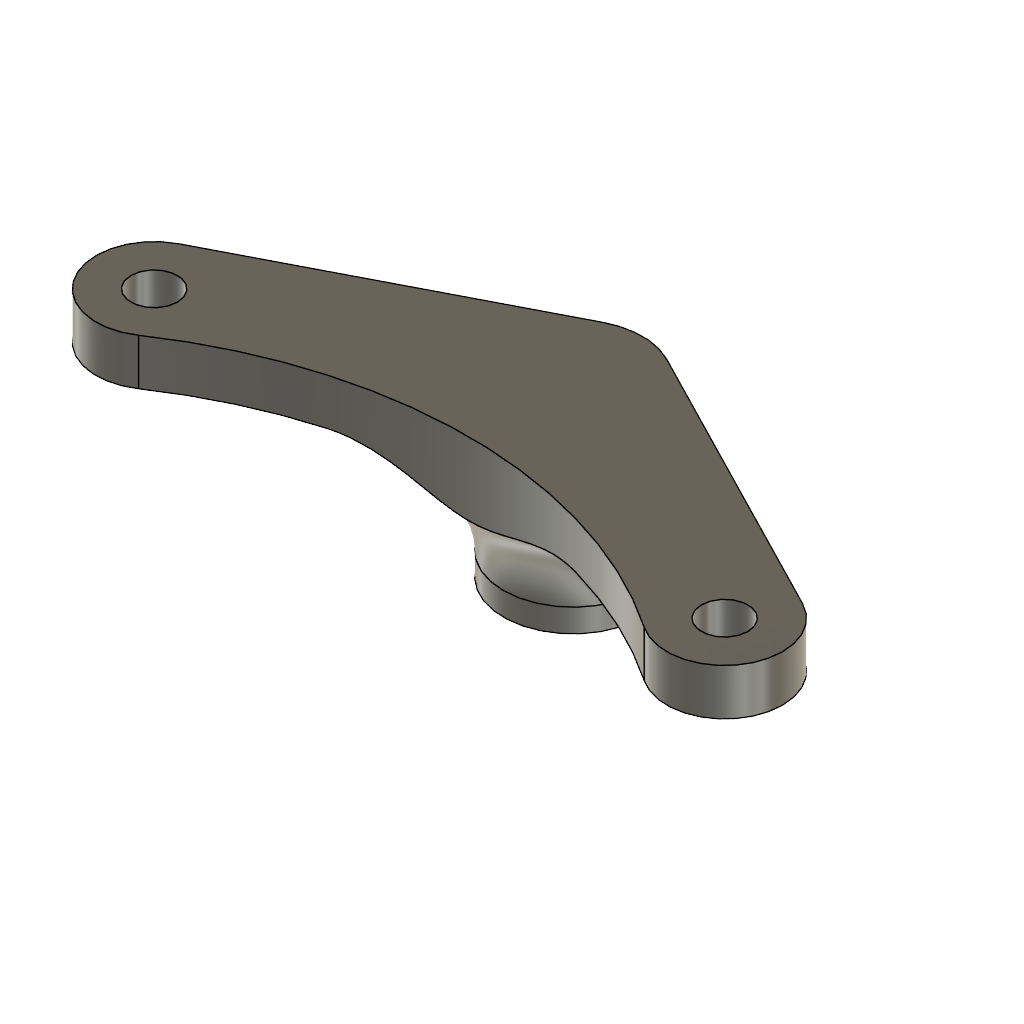
Haltebrücke (Autodesk Fusion 360 design; units mm, degrees)
Autodesk Fusion 360 part; units mm, degrees
sketch "Skizze1" plane through (0, 0, 0) normal (0, 0, 1) x (1, 0, 0)
  circle A0 centre (0, 0) radius 22 construction
  circle A1 centre (-12.3022, 18.2388) radius 1
  circle A2 centre (12.3022, 18.2388) radius 1
  line L0 (0, 0) -> (0, 38.9459) construction
  line L1 (0, 0) -> (-12.3022, 18.2388) construction
  line L2 (0, 0) -> (12.3022, 18.2388) construction
  circle A3 centre (-12.3022, 18.2388) radius 2.5
  circle A4 centre (12.3022, 18.2388) radius 2.5
  circle A5 centre (0, 24) radius 3
  line L3 (-1.3714, 26.6682) -> (-13.4451, 20.4623)
  line L4 (13.4451, 20.4623) -> (1.3714, 26.6682)
  arc A6 (10.9043, 16.1662) -> (-10.9043, 16.1662) centre (0, 0) ccw construction
  arc A7 (10.9043, 16.1662) -> (-10.9043, 16.1662) centre (0, 0) ccw
  point P0 (0, 24)
  dimension "d3" = 2
  dimension "d5" = 68
  dimension "d6" = 5
  dimension "d9" = 24
  dimension "d10" = 6
  dimension "d15" = 44
  dimension "d16" = 19.5
  constraint coincident A0.centre L0.start
  constraint coincident A0 A1.centre
  constraint coincident A0 A2.centre
  constraint vertical L0
  constraint coincident A1.centre L1.end
  constraint coincident A2.centre L2.end
  constraint symmetric A1.centre A2.centre L0
  constraint concentric A1 A3
  constraint concentric A2 A4
  constraint equal A1 A2
  constraint equal A3 A4
  constraint coincident L0 P0
  constraint coincident P0 A5.centre
  constraint coincident A5 L3.start
  constraint coincident A3 L3.end
  constraint coincident A4 L4.start
  constraint coincident A5 L4.end
  constraint tangent A5 L4
  constraint tangent A5 L3
  constraint tangent A3 L3
  constraint tangent A4 L4
  constraint concentric A0 A7
  constraint coincident L1 A6.end
  constraint coincident L2 A6.start
  constraint tangent A3 A6
  measures "d3" diameter of A1
  measures "d5" angle of L1 L2
  measures "d6" diameter of A3
  measures "d9" distance of A0.centre P0
  measures "d10" diameter of A5
  measures "d15" diameter of A0
  measures "d16" radius of A7
extrude "Extrusion1" add sketch "Skizze1" along normal blind 2
extrude "Extrusion2" add sketch "Skizze1" against normal blind 5.5 contours A5
fillet "Abrundung1" radius 4.5 1 edges at (0, 21, 0)
